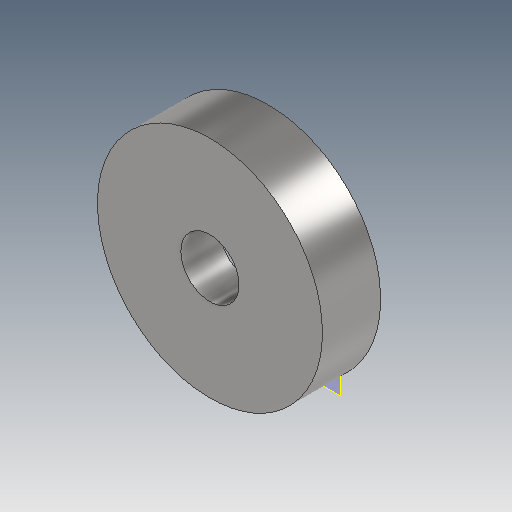
# Autodesk Inventor part: Housing of planetary gearbox part 2
Saved by Autodesk Inventor 2020.3 (Build 243373010, 373A)
## iProperties
Created: 2021-05-05
Part Number: Housing of planetary gearbox part 2
Material: Steel, Alloy
Document SubType Name: Modeling
Designer: marti
Density: 7.73 g/cm^3
Appearance: Semi-Polished
Author: marti
Autodesk Inventor part; units mm, degrees
ref_plane "YZ Plane" through (0, 0, 0) normal (1, 0, 0) x (0, 1, 0)
ref_plane "XZ Plane" through (0, 0, 0) normal (0, 1, 0) x (-1, 0, 0)
ref_plane "XY Plane" through (0, 0, 0) normal (0, 0, 1) x (1, 0, 0)
sketch "Sketch1" plane through (0, 0, 0) normal (0, 0, 1) x (1, 0, 0)
  circle A0 centre (0, 0) radius 24
  circle A1 centre (0, 0) radius 22.6875
  dimension "d0" = 48
  dimension "d2" = 45.375
  constraints: 2 centre point, 2 coincident
  measures "d0" diameter of A0
  measures "d2" diameter of A1
extrude "Extrusion1" add sketch "Sketch1" along normal blind 5
sketch "Sketch2" plane through (0, 0, 5) normal (0, 0, 1) x (1, 0, 0)
  circle A0 centre (0, 0) radius 24 projected
extrude "Extrusion2" add sketch "Sketch2" along normal blind 10
sketch "Sketch3" plane through (0, 0, 0) normal (0, 0, -1) x (-1, 0, 0)
  circle A0 centre (0, 0) radius 22.6875
  circle A1 centre (0, 0) radius 24
  arc A2 (8.8161, 21.2839) -> (-8.8161, 21.2839) centre (0, 0) ccw
  arc A3 (9.0505, 21.8498) -> (-9.0505, 21.8498) centre (0, 0) ccw
  circle A4 centre (0, 0) radius 7.5
  line L0 (0, 0) -> (0, 19.001)
  line L1 (-8.8161, 21.2839) -> (-9.0505, 21.8498)
  line L2 (8.8161, 21.2839) -> (9.0505, 21.8498)
  arc A5 (-21.2839, 8.8161) -> (-21.2839, -8.8161) centre (0, 0) ccw
  arc A6 (-21.8498, 9.0505) -> (-21.8498, -9.0505) centre (0, 0) ccw
  line L3 (-21.2839, -8.8161) -> (-21.8498, -9.0505)
  line L4 (-21.2839, 8.8161) -> (-21.8498, 9.0505)
  arc A7 (-8.8161, -21.2839) -> (8.8161, -21.2839) centre (0, 0) ccw
  arc A8 (-9.0505, -21.8498) -> (9.0505, -21.8498) centre (0, 0) ccw
  line L5 (8.8161, -21.2839) -> (9.0505, -21.8498)
  line L6 (-8.8161, -21.2839) -> (-9.0505, -21.8498)
  arc A9 (21.2839, -8.8161) -> (21.2839, 8.8161) centre (0, 0) ccw
  arc A10 (21.8498, -9.0505) -> (21.8498, 9.0505) centre (0, 0) ccw
  line L7 (21.2839, 8.8161) -> (21.8498, 9.0505)
  line L8 (21.2839, -8.8161) -> (21.8498, -9.0505)
  point P0 (-19.001, 0)
  point P1 (0, -19.001)
  point P2 (19.001, 0)
  dimension "d11" = 0.35
  dimension "d10" = 0.35
  dimension "d9" = 360
  constraints: 18 end point, 16 point on circle, 11 centre point, 2 coincident, 1 vertical, 47 other
  measures "d11" radial gap between concentric circles of A0 A2
  measures "d10" radial gap between concentric circles of A1 A3
ref_plane "Work Plane1" through (0, -22.4669, -8.75) normal (0, 0, -1) x (-1, 0, 0)
extrude "Extrusion6" cut sketch "Sketch3" against normal blind 10 contours A2 L1 A3 L2 | A5 L3 A6 L4 | A7 L5 A8 L6 | A9 L7 A10 L8
sketch "Sketch6" plane through (0, 0, 15) normal (0, 0, 1) x (1, 0, 0)
  circle A0 centre (0, 0) radius 7.5
  dimension "d29" = 15
  constraints: 1 centre point, 1 coincident
  measures "d29" diameter of A0
extrude "Extrusion7" cut sketch "Sketch6" against normal blind 10
sketch "Sketch7" plane through (0, 0, 5) normal (0, 0, -1) x (-1, 0, 0)
  circle A0 centre (0, 0) radius 7.5493
  line L0 (-4.0263, 15.0987) -> (-4.0263, 7.5493)
  arc A1 (-4.0263, 7.5493) -> (-8.5511, -0.2878) centre (0, 0) ccw
  line L1 (-8.5511, -0.2878) -> (-15.089, -4.0625)
  arc A2 (-15.089, -4.0625) -> (-11.0627, -11.0362) centre (-13.0758, -7.5493) ccw
  line L2 (-11.0627, -11.0362) -> (-4.5248, -7.2616)
  arc A3 (-4.5248, -7.2616) -> (4.5248, -7.2616) centre (0, 0) ccw
  line L3 (4.5248, -7.2616) -> (11.0627, -11.0362)
  arc A4 (11.0627, -11.0362) -> (15.089, -4.0625) centre (13.0758, -7.5493) ccw
  line L4 (15.089, -4.0625) -> (8.5511, -0.2878)
  arc A5 (8.5511, -0.2878) -> (4.0263, 7.5493) centre (0, 0) ccw
  line L5 (4.0263, 7.5493) -> (4.0263, 15.0987)
  arc A6 (4.0263, 15.0987) -> (-4.0263, 15.0987) centre (0, 15.0987) ccw
  circle A7 centre (0, 0) radius 19.125
  circle A8 centre (0, 0) radius 7.5 projected
  circle A9 centre (0, 0) radius 22.6875 projected
  dimension "d34" = 38.25
  constraints: 12 end point, 12 point on circle, 8 centre point, 1 coincident
  measures "d34" diameter of A7
extrude "Extrusion8" add sketch "Sketch7" along normal blind 2.5 contours A9
sketch "Sketch8" plane through (0, 0, 15) normal (0, 0, 1) x (1, 0, 0)
  circle A0 centre (0, 0) radius 29
  circle A1 centre (0, 0) radius 24 projected
  dimension "d35" = 58
  constraints: 1 centre point, 1 coincident
  measures "d35" diameter of A0
extrude "Extrusion9" add sketch "Sketch8" against normal up to surface (15 mm away)
sketch "Sketch9" plane through (0, 0, 0) normal (0, 0, -1) x (-1, 0, 0)
  line L0 (16.0425, 16.0425) -> (18.2743, 18.2743)
  line L1 (0, 0) -> (49.853, 0) construction
  circle A0 centre (0, 0) radius 22.6875 projected
  circle A1 centre (0, 0) radius 29 projected
  circle A2 centre (0, 0) radius 25.8438
  point P0 (-18.2743, 18.2743)
  point P1 (-18.2743, -18.2743)
  point P2 (18.2743, -18.2743)
  dimension "d39" = 45.375
  dimension "d41" = 51.6875
  dimension "d38" = 45
  dimension "d40" = 58
  dimension "d44" = 360
  dimension "d53" = 6.3125
  constraints: 4 end point, 1 coincident, 1 horizontal, 10 other
  measures "d38" angle of L1 L0
  measures "d40" diameter of A1
hole "Hole1" at (-18.2743, 18.2743, 0) at (18.2743, 18.2743, 0) at (18.2743, -18.2743, 0) at (-18.2743, -18.2743, 0) direction (0, 0, 1) diameter 2.459 depth 8.8 thread size "M3x0.5" class "6H" standard "ISO Metric profile"
sketch "Sketch10" plane through (0, 0, 0) normal (0, 0, -1) x (-1, 0, 0)
  circle A0 centre (18.2743, 18.2743) radius 1.2295 projected
  circle A1 centre (18.2743, -18.2743) radius 1.2295 projected
  circle A2 centre (-18.2743, -18.2743) radius 1.2295 projected
  circle A3 centre (-18.2743, 18.2743) radius 1.2295 projected
  point P0 (0, 0)
equation "\"d41\" = 0.5 * d40 + 0.5 * d39"
body "Solid1"
